Autodesk Fusion 360 part; units mm, degrees
(part 5 of 6)
  spline S16 degree 5 poles (-30.3241, -15.2327) (-30.3143, -15.242) (-30.2946, -15.2602) (-30.2642, -15.2865) (-30.2223, -15.3199) (-30.1678, -15.3592) (-30.1119, -15.3967) (-30.0551, -15.4332) (-29.9978, -15.4692) (-29.9401, -15.5048) (-29.8821, -15.5399) (-29.8236, -15.5744) (-29.7646, -15.6082) (-29.7048, -15.6412) (-29.6444, -15.6732) (-29.5834, -15.7045) (-29.5218, -15.735) (-29.4598, -15.765) (-29.3974, -15.7944) (-29.3347, -15.8233) (-29.2716, -15.8518) (-29.2081, -15.8797) (-29.1443, -15.907) (-29.08, -15.9338) (-29.0153, -15.96) (-28.9503, -15.9856) (-28.8849, -16.0108) (-28.8192, -16.0354) (-28.7532, -16.0595) (-28.6869, -16.0832) (-28.6202, -16.1064) (-28.5533, -16.1291) (-28.4861, -16.1513) (-28.4185, -16.1731) (-28.3507, -16.1943) (-28.2826, -16.2151) (-28.2142, -16.2355) (-28.1455, -16.2554) (-28.0766, -16.2748) (-28.0074, -16.2938) (-27.938, -16.3123) (-27.8683, -16.3304) (-27.7984, -16.3481) (-27.7282, -16.3653) (-27.6578, -16.3821) (-27.5872, -16.3984) (-27.5163, -16.4143) (-27.4452, -16.4298) (-27.3739, -16.4449) (-27.3024, -16.4595) (-27.2307, -16.4737) (-27.1587, -16.4875) (-27.0865, -16.5009) (-27.0142, -16.5139) (-26.9416, -16.5264) (-26.8689, -16.5386) (-26.7959, -16.5503) (-26.7228, -16.5616) (-26.6494, -16.5725) (-26.5759, -16.583) (-26.5022, -16.5931) (-26.4283, -16.6028) (-26.3543, -16.6121) (-26.2801, -16.621) (-26.2057, -16.6295) (-26.1311, -16.6376) (-26.0564, -16.6453) (-25.9815, -16.6526) (-25.9065, -16.6595) (-25.8313, -16.666) (-25.7559, -16.6721) (-25.6955, -16.6767) (-25.6501, -16.68) (-25.6199, -16.6821) (-25.6047, -16.6831) knots 0 0 0 0 0 0 0.01428571 0.02857143 0.04285714 0.05714286 0.07142857 0.08571429 0.1 0.11428571 0.12857143 0.14285714 0.15714286 0.17142857 0.18571429 0.2 0.21428571 0.22857143 0.24285714 0.25714286 0.27142857 0.28571429 0.3 0.31428571 0.32857143 0.34285714 0.35714286 0.37142857 0.38571429 0.4 0.41428571 0.42857143 0.44285714 0.45714286 0.47142857 0.48571429 0.5 0.51428571 0.52857143 0.54285714 0.55714286 0.57142857 0.58571429 0.6 0.61428571 0.62857143 0.64285714 0.65714286 0.67142857 0.68571429 0.7 0.71428571 0.72857143 0.74285714 0.75714286 0.77142857 0.78571429 0.8 0.81428571 0.82857143 0.84285714 0.85714286 0.87142857 0.88571429 0.9 0.91428571 0.92857143 0.94285714 0.95714286 0.97142857 0.98571429 1 1 1 1 1 1
  arc A32 (-25.6047, -16.6831) -> (-24.4732, -15.15) centre (-45.4614, -0.8441) ccw
  spline S17 degree 5 poles (-24.4732, -15.15) (-24.4787, -15.1359) (-24.4896, -15.1075) (-24.5061, -15.0651) (-24.5283, -15.0088) (-24.5564, -14.9386) (-24.5847, -14.8686) (-24.6135, -14.799) (-24.6425, -14.7296) (-24.6719, -14.6604) (-24.7016, -14.5916) (-24.7317, -14.523) (-24.762, -14.4547) (-24.7927, -14.3866) (-24.8238, -14.3189) (-24.8552, -14.2515) (-24.8869, -14.1843) (-24.9189, -14.1175) (-24.9513, -14.0509) (-24.984, -13.9846) (-25.017, -13.9187) (-25.0504, -13.8531) (-25.0841, -13.7877) (-25.1182, -13.7227) (-25.1526, -13.658) (-25.1873, -13.5937) (-25.2224, -13.5296) (-25.2578, -13.4659) (-25.2935, -13.4025) (-25.3296, -13.3395) (-25.3661, -13.2768) (-25.4029, -13.2145) (-25.44, -13.1525) (-25.4775, -13.0909) (-25.5153, -13.0297) (-25.5535, -12.9688) (-25.592, -12.9083) (-25.6309, -12.8481) (-25.6701, -12.7884) (-25.7097, -12.729) (-25.7497, -12.6701) (-25.79, -12.6115) (-25.8307, -12.5534) (-25.8718, -12.4957) (-25.9132, -12.4385) (-25.955, -12.3816) (-25.9971, -12.3252) (-26.0397, -12.2692) (-26.0826, -12.2137) (-26.1259, -12.1586) (-26.1695, -12.1041) (-26.2136, -12.05) (-26.2582, -11.9965) (-26.3031, -11.9435) (-26.3485, -11.8911) (-26.3942, -11.8392) (-26.4404, -11.7878) (-26.4869, -11.7368) (-26.5338, -11.6864) (-26.5811, -11.6366) (-26.629, -11.5875) (-26.6774, -11.5392) (-26.7265, -11.4918) (-26.7762, -11.4453) (-26.8265, -11.3996) (-26.8771, -11.3546) (-26.9281, -11.3099) (-26.9793, -11.2658) (-27.031, -11.2222) (-27.0834, -11.1799) (-27.137, -11.1394) (-27.1812, -11.1092) (-27.2153, -11.0879) (-27.2385, -11.0744) (-27.2502, -11.0678) knots -1 -1 -1 -1 -1 -1 -0.98571429 -0.97142857 -0.95714286 -0.94285714 -0.92857143 -0.91428571 -0.9 -0.88571429 -0.87142857 -0.85714286 -0.84285714 -0.82857143 -0.81428571 -0.8 -0.78571429 -0.77142857 -0.75714286 -0.74285714 -0.72857143 -0.71428571 -0.7 -0.68571429 -0.67142857 -0.65714286 -0.64285714 -0.62857143 -0.61428571 -0.6 -0.58571429 -0.57142857 -0.55714286 -0.54285714 -0.52857143 -0.51428571 -0.5 -0.48571429 -0.47142857 -0.45714286 -0.44285714 -0.42857143 -0.41428571 -0.4 -0.38571429 -0.37142857 -0.35714286 -0.34285714 -0.32857143 -0.31428571 -0.3 -0.28571429 -0.27142857 -0.25714286 -0.24285714 -0.22857143 -0.21428571 -0.2 -0.18571429 -0.17142857 -0.15714286 -0.14285714 -0.12857143 -0.11428571 -0.1 -0.08571429 -0.07142857 -0.05714286 -0.04285714 -0.02857143 -0.01428571 0 0 0 0 0 0
  line L19 (-27.2502, -11.0678) -> (-28.1194, -10.5793)
  arc A33 (-28.7833, -8.5309) -> (-28.1194, -10.5793) centre (-27.3416, -9.1954) ccw
  arc A34 (-28.7833, -8.5309) -> (-28.4826, -7.8417) centre (-45.4614, -0.8441) ccw
  arc A35 (-26.5294, -6.9351) -> (-28.4826, -7.8417) centre (-27.0149, -8.4466) ccw
  line L20 (-26.5294, -6.9351) -> (-25.5802, -7.24)
  spline S18 degree 5 poles (-25.5802, -7.24) (-25.5674, -7.2441) (-25.5417, -7.2519) (-25.5029, -7.2625) (-25.4506, -7.2743) (-25.3845, -7.2861) (-25.3178, -7.2957) (-25.2508, -7.3039) (-25.1836, -7.3115) (-25.1162, -7.3185) (-25.0487, -7.325) (-24.981, -7.3307) (-24.9131, -7.3356) (-24.845, -7.3393) (-24.7767, -7.342) (-24.7081, -7.3436) (-24.6394, -7.3444) (-24.5705, -7.3445) (-24.5016, -7.344) (-24.4325, -7.3428) (-24.3633, -7.3411) (-24.294, -7.3387) (-24.2246, -7.3356) (-24.1551, -7.3318) (-24.0855, -7.3274) (-24.0158, -7.3223) (-23.946, -7.3165) (-23.8761, -7.3102) (-23.8061, -7.3033) (-23.7361, -7.2959) (-23.666, -7.2878) (-23.5958, -7.2793) (-23.5256, -7.2701) (-23.4553, -7.2604) (-23.385, -7.2501) (-23.3146, -7.2393) (-23.2442, -7.228) (-23.1737, -7.2161) (-23.1031, -7.2037) (-23.0326, -7.1908) (-22.962, -7.1774) (-22.8914, -7.1635) (-22.8207, -7.149) (-22.75, -7.1341) (-22.6793, -7.1187) (-22.6086, -7.1027) (-22.5378, -7.0863) (-22.467, -7.0694) (-22.3962, -7.0521) (-22.3254, -7.0342) (-22.2546, -7.0159) (-22.1838, -6.9971) (-22.113, -6.9779) (-22.0422, -6.9581) (-21.9714, -6.938) (-21.9005, -6.9173) (-21.8297, -6.8962) (-21.7589, -6.8747) (-21.6881, -6.8527) (-21.6173, -6.8303) (-21.5465, -6.8074) (-21.4758, -6.7841) (-21.405, -6.7603) (-21.3343, -6.7361) (-21.2636, -6.7115) (-21.1929, -6.6865) (-21.1222, -6.661) (-21.0516, -6.6351) (-20.981, -6.6087) (-20.9104, -6.582) (-20.8399, -6.5548) (-20.7834, -6.5327) (-20.7412, -6.516) (-20.713, -6.5047) (-20.6989, -6.4991) knots 0 0 0 0 0 0 0.01428571 0.02857143 0.04285714 0.05714286 0.07142857 0.08571429 0.1 0.11428571 0.12857143 0.14285714 0.15714286 0.17142857 0.18571429 0.2 0.21428571 0.22857143 0.24285714 0.25714286 0.27142857 0.28571429 0.3 0.31428571 0.32857143 0.34285714 0.35714286 0.37142857 0.38571429 0.4 0.41428571 0.42857143 0.44285714 0.45714286 0.47142857 0.48571429 0.5 0.51428571 0.52857143 0.54285714 0.55714286 0.57142857 0.58571429 0.6 0.61428571 0.62857143 0.64285714 0.65714286 0.67142857 0.68571429 0.7 0.71428571 0.72857143 0.74285714 0.75714286 0.77142857 0.78571429 0.8 0.81428571 0.82857143 0.84285714 0.85714286 0.87142857 0.88571429 0.9 0.91428571 0.92857143 0.94285714 0.95714286 0.97142857 0.98571429 1 1 1 1 1 1
  arc A36 (-20.6989, -6.4991) -> (-20.3446, -4.6269) centre (-45.4614, -0.8441) ccw
  spline S19 degree 5 poles (-20.3446, -4.6269) (-20.3557, -4.6165) (-20.3778, -4.5957) (-20.4111, -4.5647) (-20.4555, -4.5235) (-20.5113, -4.4724) (-20.5672, -4.4217) (-20.6233, -4.3714) (-20.6796, -4.3215) (-20.736, -4.272) (-20.7927, -4.2228) (-20.8495, -4.1741) (-20.9065, -4.1257) (-20.9637, -4.0777) (-21.0211, -4.0302) (-21.0786, -3.983) (-21.1363, -3.9363) (-21.1942, -3.8899) (-21.2522, -3.844) (-21.3104, -3.7985) (-21.3688, -3.7534) (-21.4274, -3.7088) (-21.4861, -3.6645) (-21.545, -3.6208) (-21.604, -3.5774) (-21.6633, -3.5345) (-21.7226, -3.492) (-21.7822, -3.45) (-21.8419, -3.4084) (-21.9018, -3.3673) (-21.9618, -3.3266) (-22.022, -3.2864) (-22.0823, -3.2467) (-22.1428, -3.2074) (-22.2035, -3.1686) (-22.2643, -3.1304) (-22.3253, -3.0926) (-22.3864, -3.0553) (-22.4477, -3.0185) (-22.5091, -2.9822) (-22.5707, -2.9464) (-22.6324, -2.9111) (-22.6943, -2.8764) (-22.7563, -2.8422) (-22.8185, -2.8086) (-22.8808, -2.7755) (-22.9433, -2.743) (-23.0059, -2.711) (-23.0686, -2.6796) (-23.1315, -2.6488) (-23.1945, -2.6186) (-23.2577, -2.589) (-23.3211, -2.5601) (-23.3845, -2.5319) (-23.4482, -2.5043) (-23.5119, -2.4774) (-23.5758, -2.4511) (-23.6398, -2.4254) (-23.7039, -2.4003) (-23.7682, -2.376) (-23.8326, -2.3525) (-23.8972, -2.33) (-23.962, -2.3086) (-24.0269, -2.2883) (-24.092, -2.2689) (-24.1572, -2.2503) (-24.2225, -2.2322) (-24.2879, -2.2147) (-24.3533, -2.1978) (-24.4189, -2.1824) (-24.4847, -2.1692) (-24.5377, -2.1611) (-24.5777, -2.1568) (-24.6044, -2.1547) (-24.6178, -2.1539) knots -1 -1 -1 -1 -1 -1 -0.98571429 -0.97142857 -0.95714286 -0.94285714 -0.92857143 -0.91428571 -0.9 -0.88571429 -0.87142857 -0.85714286 -0.84285714 -0.82857143 -0.81428571 -0.8 -0.78571429 -0.77142857 -0.75714286 -0.74285714 -0.72857143 -0.71428571 -0.7 -0.68571429 -0.67142857 -0.65714286 -0.64285714 -0.62857143 -0.61428571 -0.6 -0.58571429 -0.57142857 -0.55714286 -0.54285714 -0.52857143 -0.51428571 -0.5 -0.48571429 -0.47142857 -0.45714286 -0.44285714 -0.42857143 -0.41428571 -0.4 -0.38571429 -0.37142857 -0.35714286 -0.34285714 -0.32857143 -0.31428571 -0.3 -0.28571429 -0.27142857 -0.25714286 -0.24285714 -0.22857143 -0.21428571 -0.2 -0.18571429 -0.17142857 -0.15714286 -0.14285714 -0.12857143 -0.11428571 -0.1 -0.08571429 -0.07142857 -0.05714286 -0.04285714 -0.02857143 -0.01428571 0 0 0 0 0 0
  line L21 (-24.6178, -2.1539) -> (-25.6129, -2.0908)
  arc A37 (-27.0998, -0.5334) -> (-25.6129, -2.0908) centre (-25.5125, -0.5065) ccw
  arc A38 (-27.0998, -0.5334) -> (-27.1279, 0.2181) centre (-45.4614, -0.8441) ccw
  arc A39 (-25.7615, 1.8823) -> (-27.1279, 0.2181) centre (-25.5431, 0.31) ccw
  line L22 (-25.7615, 1.8823) -> (-24.774, 2.0195)
  spline S20 degree 5 poles (-24.774, 2.0195) (-24.7607, 2.0214) (-24.7342, 2.0255) (-24.6946, 2.0328) (-24.6424, 2.0448) (-24.5777, 2.0629) (-24.5135, 2.0832) (-24.4495, 2.1048) (-24.3856, 2.1272) (-24.3219, 2.1501) (-24.2583, 2.1736) (-24.1948, 2.1977) (-24.1315, 2.2228) (-24.0685, 2.249) (-24.0058, 2.2763) (-23.9433, 2.3045) (-23.8811, 2.3336) (-23.819, 2.3634) (-23.7571, 2.3938) (-23.6953, 2.4248) (-23.6338, 2.4564) (-23.5724, 2.4887) (-23.5112, 2.5216) (-23.4502, 2.5551) (-23.3894, 2.5893) (-23.3288, 2.6242) (-23.2684, 2.6596) (-23.2082, 2.6956) (-23.1481, 2.7322) (-23.0883, 2.7693) (-23.0286, 2.8069) (-22.9691, 2.8451) (-22.9098, 2.8838) (-22.8507, 2.9231) (-22.7918, 2.9628) (-22.7331, 3.0031) (-22.6745, 3.0439) (-22.6162, 3.0852) (-22.558, 3.127) (-22.5, 3.1692) (-22.4422, 3.2119) (-22.3846, 3.2551) (-22.3272, 3.2988) (-22.27, 3.3429) (-22.213, 3.3875) (-22.1562, 3.4325) (-22.0996, 3.478) (-22.0431, 3.5239) (-21.9869, 3.5703) (-21.9309, 3.6171) (-21.875, 3.6643) (-21.8194, 3.712) (-21.7639, 3.76) (-21.7086, 3.8085) (-21.6536, 3.8574) (-21.5987, 3.9068) (-21.5441, 3.9565) (-21.4896, 4.0066) (-21.4354, 4.0572) (-21.3813, 4.1081) (-21.3275, 4.1594) (-21.2739, 4.2111) (-21.2204, 4.2632) (-21.1672, 4.3157) (-21.1142, 4.3686) (-21.0613, 4.4218) (-21.0087, 4.4754) (-20.9563, 4.5294) (-20.9041, 4.5838) (-20.8522, 4.6385) (-20.8004, 4.6936) (-20.7592, 4.738) (-20.7283, 4.7714) (-20.7078, 4.7938) (-20.6975, 4.805) knots 0 0 0 0 0 0 0.01428571 0.02857143 0.04285714 0.05714286 0.07142857 0.08571429 0.1 0.11428571 0.12857143 0.14285714 0.15714286 0.17142857 0.18571429 0.2 0.21428571 0.22857143 0.24285714 0.25714286 0.27142857 0.28571429 0.3 0.31428571 0.32857143 0.34285714 0.35714286 0.37142857 0.38571429 0.4 0.41428571 0.42857143 0.44285714 0.45714286 0.47142857 0.48571429 0.5 0.51428571 0.52857143 0.54285714 0.55714286 0.57142857 0.58571429 0.6 0.61428571 0.62857143 0.64285714 0.65714286 0.67142857 0.68571429 0.7 0.71428571 0.72857143 0.74285714 0.75714286 0.77142857 0.78571429 0.8 0.81428571 0.82857143 0.84285714 0.85714286 0.87142857 0.88571429 0.9 0.91428571 0.92857143 0.94285714 0.95714286 0.97142857 0.98571429 1 1 1 1 1 1
  arc A40 (-20.6975, 4.805) -> (-21.1907, 6.6455) centre (-45.4614, -0.8441) ccw
  spline S21 degree 5 poles (-21.1907, 6.6455) (-21.2052, 6.65) (-21.2341, 6.6592) (-21.2776, 6.6727) (-21.3355, 6.6905) (-21.4078, 6.7123) (-21.4802, 6.7337) (-21.5526, 6.7547) (-21.625, 6.7753) (-21.6974, 6.7954) (-21.7697, 6.8151) (-21.8421, 6.8344) (-21.9144, 6.8532) (-21.9867, 6.8716) (-22.059, 6.8896) (-22.1313, 6.9071) (-22.2036, 6.9242) (-22.2759, 6.9408) (-22.3481, 6.957) (-22.4203, 6.9728) (-22.4924, 6.988) (-22.5646, 7.0029) (-22.6367, 7.0172) (-22.7087, 7.0312) (-22.7807, 7.0446) (-22.8527, 7.0576) (-22.9247, 7.0701) (-22.9965, 7.0821) (-23.0684, 7.0937) (-23.1402, 7.1047) (-23.2119, 7.1153) (-23.2836, 7.1254) (-23.3552, 7.135) (-23.4267, 7.1442) (-23.4982, 7.1528) (-23.5696, 7.1609) (-23.6409, 7.1685) (-23.7122, 7.1756) (-23.7833, 7.1821) (-23.8544, 7.1882) (-23.9254, 7.1937) (-23.9964, 7.1987) (-24.0672, 7.2031) (-24.1379, 7.207) (-24.2085, 7.2103) (-24.279, 7.2131) (-24.3494, 7.2153) (-24.4197, 7.2169) (-24.4898, 7.218) (-24.5599, 7.2185) (-24.6298, 7.2184) (-24.6995, 7.2176) (-24.7691, 7.2162) (-24.8385, 7.214) (-24.9078, 7.2113) (-24.9769, 7.2078) (-25.0459, 7.2038) (-25.1147, 7.1992) (-25.1834, 7.194) (-25.2519, 7.1881) (-25.3201, 7.1813) (-25.3881, 7.1735) (-25.4557, 7.1647) (-25.523, 7.1548) (-25.5901, 7.144) (-25.6569, 7.1325) (-25.7236, 7.1204) (-25.7901, 7.1079) (-25.8563, 7.0947) (-25.9221, 7.0801) (-25.9871, 7.0634) (-26.0384, 7.0477) (-26.0763, 7.0343) (-26.1013, 7.0246) (-26.1137, 7.0195) knots -1 -1 -1 -1 -1 -1 -0.98571429 -0.97142857 -0.95714286 -0.94285714 -0.92857143 -0.91428571 -0.9 -0.88571429 -0.87142857 -0.85714286 -0.84285714 -0.82857143 -0.81428571 -0.8 -0.78571429 -0.77142857 -0.75714286 -0.74285714 -0.72857143 -0.71428571 -0.7 -0.68571429 -0.67142857 -0.65714286 -0.64285714 -0.62857143 -0.61428571 -0.6 -0.58571429 -0.57142857 -0.55714286 -0.54285714 -0.52857143 -0.51428571 -0.5 -0.48571429 -0.47142857 -0.45714286 -0.44285714 -0.42857143 -0.41428571 -0.4 -0.38571429 -0.37142857 -0.35714286 -0.34285714 -0.32857143 -0.31428571 -0.3 -0.28571429 -0.27142857 -0.25714286 -0.24285714 -0.22857143 -0.21428571 -0.2 -0.18571429 -0.17142857 -0.15714286 -0.14285714 -0.12857143 -0.11428571 -0.1 -0.08571429 -0.07142857 -0.05714286 -0.04285714 -0.02857143 -0.01428571 0 0 0 0 0 0
  line L23 (-26.1137, 7.0195) -> (-27.0376, 6.6446)
  arc A41 (-29.053, 7.4026) -> (-27.0376, 6.6446) centre (-27.6346, 8.1155) ccw
  arc A42 (-29.053, 7.4026) -> (-29.4044, 8.0675) centre (-45.4614, -0.8441) ccw
  arc A43 (-28.8954, 10.1598) -> (-29.4044, 8.0675) centre (-28.0164, 8.8379) ccw
  line L24 (-28.8954, 10.1598) -> (-28.0652, 10.7119)
  spline S22 degree 5 poles (-28.0652, 10.7119) (-28.054, 10.7193) (-28.0319, 10.7345) (-27.9994, 10.7582) (-27.9576, 10.7917) (-27.9071, 10.8361) (-27.8581, 10.8822) (-27.8098, 10.9295) (-27.762, 10.9774) (-27.7145, 11.0257) (-27.6674, 11.0744) (-27.6207, 11.1237) (-27.5746, 11.1738) (-27.5292, 11.2247) (-27.4845, 11.2765) (-27.4404, 11.329) (-27.397, 11.3823) (-27.354, 11.4361) (-27.3114, 11.4903) (-27.2692, 11.545) (-27.2275, 11.6002) (-27.1861, 11.6559) (-27.1453, 11.7121) (-27.1049, 11.7688) (-27.0649, 11.826) (-27.0255, 11.8837) (-26.9864, 11.9418) (-26.9478, 12.0004) (-26.9096, 12.0594) (-26.8717, 12.1188) (-26.8343, 12.1786) (-26.7973, 12.2388) (-26.7606, 12.2994) (-26.7244, 12.3604) (-26.6886, 12.4218) (-26.6531, 12.4836) (-26.6181, 12.5457) (-26.5834, 12.6082) (-26.5491, 12.6711) (-26.5152, 12.7343) (-26.4817, 12.7979) (-26.4486, 12.8618) (-26.4158, 12.926) (-26.3834, 12.9906) (-26.3514, 13.0555) (-26.3197, 13.1207) (-26.2884, 13.1863) (-26.2575, 13.2522) (-26.227, 13.3183) (-26.1968, 13.3848) (-26.1669, 13.4516) (-26.1375, 13.5187) (-26.1084, 13.586) (-26.0796, 13.6537) (-26.0513, 13.7217) (-26.0232, 13.7899) (-25.9956, 13.8584) (-25.9683, 13.9272) (-25.9413, 13.9963) (-25.9147, 14.0656) (-25.8885, 14.1352) (-25.8626, 14.2051) (-25.837, 14.2752) (-25.8118, 14.3456) (-25.787, 14.4162) (-25.7625, 14.4871) (-25.7384, 14.5582) (-25.7146, 14.6296) (-25.6912, 14.7012) (-25.6681, 14.7731) (-25.6454, 14.8452) (-25.6274, 14.9031) (-25.6142, 14.9466) (-25.6054, 14.9756) (-25.601, 14.9902) knots 0 0 0 0 0 0 0.01428571 0.02857143 0.04285714 0.05714286 0.07142857 0.08571429 0.1 0.11428571 0.12857143 0.14285714 0.15714286 0.17142857 0.18571429 0.2 0.21428571 0.22857143 0.24285714 0.25714286 0.27142857 0.28571429 0.3 0.31428571 0.32857143 0.34285714 0.35714286 0.37142857 0.38571429 0.4 0.41428571 0.42857143 0.44285714 0.45714286 0.47142857 0.48571429 0.5 0.51428571 0.52857143 0.54285714 0.55714286 0.57142857 0.58571429 0.6 0.61428571 0.62857143 0.64285714 0.65714286 0.67142857 0.68571429 0.7 0.71428571 0.72857143 0.74285714 0.75714286 0.77142857 0.78571429 0.8 0.81428571 0.82857143 0.84285714 0.85714286 0.87142857 0.88571429 0.9 0.91428571 0.92857143 0.94285714 0.95714286 0.97142857 0.98571429 1 1 1 1 1 1
  arc A44 (-25.601, 14.9902) -> (-26.8439, 16.4344) centre (-45.4614, -0.8441) ccw
  spline S23 degree 5 poles (-26.8439, 16.4344) (-26.8589, 16.4323) (-26.8889, 16.4279) (-26.9339, 16.4213) (-26.9938, 16.4122) (-27.0685, 16.4004) (-27.143, 16.3883) (-27.2173, 16.3758) (-27.2915, 16.3629) (-27.3654, 16.3497) (-27.4392, 16.336) (-27.5127, 16.322) (-27.5861, 16.3076) (-27.6592, 16.2928) (-27.7322, 16.2776) (-27.8049, 16.262) (-27.8774, 16.2461) (-27.9497, 16.2297) (-28.0218, 16.213) (-28.0937, 16.1958) (-28.1653, 16.1783) (-28.2368, 16.1603) (-28.308, 16.142) (-28.3789, 16.1233) (-28.4496, 16.1041) (-28.5201, 16.0846) (-28.5903, 16.0646) (-28.6603, 16.0443) (-28.7301, 16.0235) (-28.7996, 16.0024) (-28.8688, 15.9808) (-28.9377, 15.9588) (-29.0064, 15.9364) (-29.0748, 15.9135) (-29.143, 15.8903) (-29.2108, 15.8666) (-29.2784, 15.8425) (-29.3456, 15.818) (-29.4126, 15.793) (-29.4793, 15.7676) (-29.5457, 15.7418) (-29.6117, 15.7155) (-29.6774, 15.6888) (-29.7428, 15.6616) (-29.8079, 15.634) (-29.8726, 15.6059) (-29.937, 15.5773) (-30.001, 15.5483) (-30.0647, 15.5188) (-30.128, 15.4889) (-30.1909, 15.4584) (-30.2535, 15.4275) (-30.3155, 15.396) (-30.3772, 15.3639) (-30.4384, 15.3314) (-30.4992, 15.2983) (-30.5596, 15.2648) (-30.6196, 15.2307) (-30.6792, 15.1962) (-30.7383, 15.1612) (-30.7968, 15.1255) (-30.8547, 15.089) (-30.9118, 15.0517) (-30.9682, 15.0136) (-31.0239, 14.9747) (-31.0791, 14.9354) (-31.1339, 14.8956) (-31.1884, 14.8555) (-31.2423, 14.8148) (-31.2953, 14.7732) (-31.3467, 14.7299) (-31.386, 14.6935) (-31.4143, 14.665) (-31.4326, 14.6454) (-31.4417, 14.6354) knots -1 -1 -1 -1 -1 -1 -0.98571429 -0.97142857 -0.95714286 -0.94285714 -0.92857143 -0.91428571 -0.9 -0.88571429 -0.87142857 -0.85714286 -0.84285714 -0.82857143 -0.81428571 -0.8 -0.78571429 -0.77142857 -0.75714286 -0.74285714 -0.72857143 -0.71428571 -0.7 -0.68571429 -0.67142857 -0.65714286 -0.64285714 -0.62857143 -0.61428571 -0.6 -0.58571429 -0.57142857 -0.55714286 -0.54285714 -0.52857143 -0.51428571 -0.5 -0.48571429 -0.47142857 -0.45714286 -0.44285714 -0.42857143 -0.41428571 -0.4 -0.38571429 -0.37142857 -0.35714286 -0.34285714 -0.32857143 -0.31428571 -0.3 -0.28571429 -0.27142857 -0.25714286 -0.24285714 -0.22857143 -0.21428571 -0.2 -0.18571429 -0.17142857 -0.15714286 -0.14285714 -0.12857143 -0.11428571 -0.1 -0.08571429 -0.07142857 -0.05714286 -0.04285714 -0.02857143 -0.01428571 0 0 0 0 0 0
  line L25 (-31.4417, 14.6354) -> (-32.1113, 13.8967)
  arc A45 (-34.2561, 13.7053) -> (-32.1113, 13.8967) centre (-33.2874, 14.963) ccw
  arc A46 (-34.2561, 13.7053) -> (-34.8612, 14.1518) centre (-45.4614, -0.8441) ccw
  arc A47 (-35.3981, 14.8093) -> (-34.8612, 14.1518) centre (-33.9448, 15.4482) ccw
  line L26 (-35.3981, 14.8093) -> (-33.2667, 19.4605)
  line L27 (-33.2667, 19.4605) -> (-34.2844, 20.5142)
  spline S24 degree 5 poles (-34.2844, 20.5142) (-34.2847, 20.5222) (-34.2856, 20.5448) (-34.2873, 20.5821) (-34.2898, 20.6341) (-34.2933, 20.7009) (-34.2977, 20.7746) (-34.3025, 20.8483) (-34.3077, 20.9221) (-34.3134, 20.996) (-34.3195, 21.0701) (-34.3261, 21.1441) (-34.3331, 21.2183) (-34.3405, 21.2926) (-34.3483, 21.3669) (-34.3566, 21.4413) (-34.3653, 21.5158) (-34.3744, 21.5904) (-34.384, 21.665) (-34.3939, 21.7397) (-34.4043, 21.8145) (-34.4151, 21.8893) (-34.4241, 21.9492) (-34.431, 21.9942) (-34.4357, 22.0242) (-34.4381, 22.0392) knots 0.70654 0.70654 0.70654 0.70654 0.70654 0.70654 0.714286 0.728571 0.742857 0.757143 0.771429 0.785714 0.8 0.814286 0.828571 0.842857 0.857143 0.871429 0.885714 0.9 0.914286 0.928571 0.942857 0.957143 0.971429 0.985714 1 1 1 1 1 1
  arc A48 (-34.4381, 22.0392) -> (-36.1845, 22.8011) centre (-45.4614, -0.8441) ccw
  spline S25 degree 5 poles (-36.1845, 22.8011) (-36.1971, 22.7927) (-36.2223, 22.7757) (-36.2596, 22.7504) (-36.2968, 22.725) (-36.3338, 22.6995) (-36.3583, 22.6825) (-36.3704, 22.6741) knots -1 -1 -1 -1 -1 -1 -0.985714 -0.971429 -0.957523 -0.957523 -0.957523 -0.957523 -0.957523 -0.957523
  line L28 (-36.3704, 22.6741) -> (-49.1726, 35.9298)
  line L29 (-49.1726, 35.9298) -> (-55.9036, 35.9298)
  line L30 (-49.1726, 17.3449) -> (-49.1726, 18.5703)
  line L31 (-49.1726, 18.5703) -> (-48.6457, 18.4228)
  arc A49 (-49.1726, 17.3449) -> (-48.6457, 18.4228) centre (-50.2296, 18.5294) ccw
  circle A50 centre (-45.4614, -0.8441) radius 3.175
  dimension "d39" = 6.35
  constraint concentric A0 A50
  measures "d39" diameter of A50
extrude "Extrude6" cut sketch "Sketch15" against normal blind 15.24 contours A50 sketch seen with x (0.965926, -0.258819, 0) y (0.258819, 0.965926, 0) z (0, 0, 1) at (44.1308, -10.9509, 0) bodies 2 in component "Spur Gear (14 teeth) (1)"
sketch "Sketch16" plane through (0, 0, 12.7) normal (0, 0, 1) x (1, 0, 0)
  circle A0 centre (-45.4614, -0.8441) radius 3.175
  line L0 (-55.9036, 35.9298) -> (-55.9036, 101.81)
  line L1 (-55.9036, 101.81) -> (-55.9735, 101.81)
  line L2 (-55.9735, 101.81) -> (-55.9735, 21.7403)
  spline S0 degree 5 poles (-55.9735, 21.7403) (-55.9837, 21.7467) (-56.0067, 21.761) (-56.0426, 21.7832) (-56.0913, 21.8132) (-56.1531, 21.8508) (-56.2177, 21.8896) (-56.2826, 21.928) (-56.3479, 21.9663) (-56.4003, 21.9966) (-56.4398, 22.0192) (-56.4661, 22.0343) (-56.4794, 22.0418) knots 0.888467 0.888467 0.888467 0.888467 0.888467 0.888467 0.9 0.914286 0.928571 0.942857 0.957143 0.971429 0.985714 1 1 1 1 1 1
  arc A1 (-56.4794, 22.0418) -> (-58.1639, 21.1514) centre (-45.4614, -0.8441) ccw
  spline S1 degree 5 poles (-58.1639, 21.1514) (-58.1652, 21.1363) (-58.1676, 21.106) (-58.1712, 21.0607) (-58.1756, 21.0003) (-58.1808, 20.9248) (-58.1856, 20.8495) (-58.1899, 20.7743) (-58.1939, 20.6991) (-58.1974, 20.6241) (-58.2005, 20.5492) (-58.2032, 20.4743) (-58.2055, 20.3996) (-58.2073, 20.325) (-58.2087, 20.2505) (-58.2097, 20.1761) (-58.2103, 20.1019) (-58.2104, 20.0277) (-58.2101, 19.9537) (-58.2094, 19.8798) (-58.2083, 19.8061) (-58.2067, 19.7325) (-58.2046, 19.659) (-58.2022, 19.5856) (-58.1992, 19.5124) (-58.1959, 19.4394) (-58.1921, 19.3665) (-58.1878, 19.2937) (-58.1831, 19.2211) (-58.1779, 19.1486) (-58.1723, 19.0763) (-58.1662, 19.0042) (-58.1596, 18.9323) (-58.1526, 18.8605) (-58.1451, 18.7889) (-58.1371, 18.7175) (-58.1286, 18.6463) (-58.1197, 18.5752) (-58.1102, 18.5044) (-58.1003, 18.4337) (-58.0899, 18.3632) (-58.079, 18.293) (-58.0675, 18.223) (-58.0556, 18.1532) (-58.0431, 18.0836) (-58.0301, 18.0143) (-58.0166, 17.9451) (-58.0026, 17.8763) (-57.988, 17.8076) (-57.9729, 17.7392) (-57.9572, 17.6711) (-57.941, 17.6033) (-57.9241, 17.5357) (-57.9065, 17.4685) (-57.8884, 17.4016) (-57.8697, 17.335) (-57.8504, 17.2686) (-57.8306, 17.2025) (-57.8103, 17.1368) (-57.7892, 17.0713) (-57.7674, 17.0063) (-57.7447, 16.9418) (-57.7211, 16.8778) (-57.6965, 16.8144) (-57.671, 16.7514) (-57.6449, 16.6888) (-57.6183, 16.6265) (-57.5913, 16.5645) (-57.5637, 16.5029) (-57.5349, 16.442) (-57.5041, 16.3822) (-57.4774, 16.3358) (-57.4559, 16.3018) (-57.4408, 16.2796) (-57.4332, 16.2686) knots -1 -1 -1 -1 -1 -1 -0.98571429 -0.97142857 -0.95714286 -0.94285714 -0.92857143 -0.91428571 -0.9 -0.88571429 -0.87142857 -0.85714286 -0.84285714 -0.82857143 -0.81428571 -0.8 -0.78571429 -0.77142857 -0.75714286 -0.74285714 -0.72857143 -0.71428571 -0.7 -0.68571429 -0.67142857 -0.65714286 -0.64285714 -0.62857143 -0.61428571 -0.6 -0.58571429 -0.57142857 -0.55714286 -0.54285714 -0.52857143 -0.51428571 -0.5 -0.48571429 -0.47142857 -0.45714286 -0.44285714 -0.42857143 -0.41428571 -0.4 -0.38571429 -0.37142857 -0.35714286 -0.34285714 -0.32857143 -0.31428571 -0.3 -0.28571429 -0.27142857 -0.25714286 -0.24285714 -0.22857143 -0.21428571 -0.2 -0.18571429 -0.17142857 -0.15714286 -0.14285714 -0.12857143 -0.11428571 -0.1 -0.08571429 -0.07142857 -0.05714286 -0.04285714 -0.02857143 -0.01428571 0 0 0 0 0 0
  line L3 (-57.4332, 16.2686) -> (-56.862, 15.4514)
  arc A2 (-57.1526, 13.3178) -> (-56.862, 15.4514) centre (-58.1632, 14.542) ccw
  arc A3 (-57.1526, 13.3178) -> (-57.7226, 12.8272) centre (-45.4614, -0.8441) ccw
  arc A4 (-59.8757, 12.8579) -> (-57.7226, 12.8272) centre (-58.7825, 14.009) ccw
  line L4 (-59.8757, 12.8579) -> (-60.5987, 13.5444)
  spline S2 degree 5 poles (-60.5987, 13.5444) (-60.6084, 13.5537) (-60.6281, 13.5719) (-60.6585, 13.5982) (-60.7005, 13.6316) (-60.7549, 13.6709) (-60.8109, 13.7084) (-60.8677, 13.745) (-60.925, 13.7809) (-60.9826, 13.8165) (-61.0407, 13.8516) (-61.0991, 13.8862) (-61.1582, 13.92) (-61.2179, 13.9529) (-61.2783, 13.9849) (-61.3394, 14.0162) (-61.401, 14.0467) (-61.463, 14.0767) (-61.5253, 14.1061) (-61.5881, 14.135) (-61.6512, 14.1635) (-61.7146, 14.1914) (-61.7785, 14.2187) (-61.8428, 14.2455) (-61.9074, 14.2717) (-61.9724, 14.2973) (-62.0378, 14.3225) (-62.1035, 14.3471) (-62.1695, 14.3712) (-62.2359, 14.3949) (-62.3025, 14.4181) (-62.3695, 14.4408) (-62.4367, 14.463) (-62.5042, 14.4848) (-62.5721, 14.506) (-62.6402, 14.5268) (-62.7086, 14.5472) (-62.7772, 14.5671) (-62.8461, 14.5865) (-62.9153, 14.6055) (-62.9847, 14.624) (-63.0544, 14.6421) (-63.1243, 14.6598) (-63.1945, 14.677) (-63.2649, 14.6938) (-63.3356, 14.7101) (-63.4064, 14.726) (-63.4775, 14.7415) (-63.5488, 14.7566) (-63.6204, 14.7712) (-63.6921, 14.7854) (-63.7641, 14.7992) (-63.8362, 14.8126) (-63.9086, 14.8256) (-63.9811, 14.8381) (-64.0539, 14.8503) (-64.1269, 14.862) (-64.2, 14.8733) (-64.2733, 14.8842) (-64.3468, 14.8947) (-64.4205, 14.9048) (-64.4944, 14.9145) (-64.5685, 14.9238) (-64.6427, 14.9327) (-64.7171, 14.9412) (-64.7916, 14.9493) (-64.8664, 14.957) (-64.9412, 14.9643) (-65.0163, 14.9712) (-65.0915, 14.9777) (-65.1668, 14.9838) (-65.2272, 14.9884) (-65.2726, 14.9917) (-65.3029, 14.9938) (-65.318, 14.9948) knots 0 0 0 0 0 0 0.01428571 0.02857143 0.04285714 0.05714286 0.07142857 0.08571429 0.1 0.11428571 0.12857143 0.14285714 0.15714286 0.17142857 0.18571429 0.2 0.21428571 0.22857143 0.24285714 0.25714286 0.27142857 0.28571429 0.3 0.31428571 0.32857143 0.34285714 0.35714286 0.37142857 0.38571429 0.4 0.41428571 0.42857143 0.44285714 0.45714286 0.47142857 0.48571429 0.5 0.51428571 0.52857143 0.54285714 0.55714286 0.57142857 0.58571429 0.6 0.61428571 0.62857143 0.64285714 0.65714286 0.67142857 0.68571429 0.7 0.71428571 0.72857143 0.74285714 0.75714286 0.77142857 0.78571429 0.8 0.81428571 0.82857143 0.84285714 0.85714286 0.87142857 0.88571429 0.9 0.91428571 0.92857143 0.94285714 0.95714286 0.97142857 0.98571429 1 1 1 1 1 1
  arc A5 (-65.318, 14.9948) -> (-66.4495, 13.4617) centre (-45.4614, -0.8441) ccw
  spline S3 degree 5 poles (-66.4495, 13.4617) (-66.4441, 13.4476) (-66.4331, 13.4192) (-66.4166, 13.3768) (-66.3945, 13.3205) (-66.3664, 13.2503) (-66.338, 13.1803) (-66.3093, 13.1107) (-66.2802, 13.0413) (-66.2509, 12.9721) (-66.2211, 12.9033) (-66.1911, 12.8347) (-66.1607, 12.7664) (-66.13, 12.6984) (-66.099, 12.6306) (-66.0676, 12.5632) (-66.0359, 12.496) (-66.0039, 12.4292) (-65.9715, 12.3626) (-65.9388, 12.2964) (-65.9057, 12.2304) (-65.8723, 12.1648) (-65.8386, 12.0994) (-65.8046, 12.0344) (-65.7702, 11.9697) (-65.7354, 11.9054) (-65.7004, 11.8413) (-65.665, 11.7776) (-65.6292, 11.7143) (-65.5931, 11.6512) (-65.5567, 11.5885) (-65.5199, 11.5262) (-65.4828, 11.4642) (-65.4453, 11.4026) (-65.4074, 11.3414) (-65.3693, 11.2805) (-65.3307, 11.22) (-65.2918, 11.1599) (-65.2526, 11.1001) (-65.213, 11.0408) (-65.1731, 10.9818) (-65.1327, 10.9233) (-65.0921, 10.8651) (-65.051, 10.8074) (-65.0096, 10.7502) (-64.9678, 10.6933) (-64.9256, 10.6369) (-64.8831, 10.5809) (-64.8402, 10.5254) (-64.7969, 10.4703) (-64.7532, 10.4158) (-64.7091, 10.3617) (-64.6646, 10.3082) (-64.6196, 10.2552) (-64.5743, 10.2028) (-64.5285, 10.1509) (-64.4824, 10.0995) (-64.4359, 10.0485) (-64.389, 9.9981) (-64.3416, 9.9483) (-64.2938, 9.8992) (-64.2453, 9.8509) (-64.1963, 9.8035) (-64.1466, 9.757) (-64.0963, 9.7113) (-64.0456, 9.6663) (-63.9947, 9.6217) (-63.9434, 9.5775) (-63.8918, 9.534) (-63.8394, 9.4916) (-63.7858, 9.4511) (-63.7415, 9.4209) (-63.7074, 9.3996) (-63.6842, 9.3861) (-63.6725, 9.3795) knots -1 -1 -1 -1 -1 -1 -0.98571429 -0.97142857 -0.95714286 -0.94285714 -0.92857143 -0.91428571 -0.9 -0.88571429 -0.87142857 -0.85714286 -0.84285714 -0.82857143 -0.81428571 -0.8 -0.78571429 -0.77142857 -0.75714286 -0.74285714 -0.72857143 -0.71428571 -0.7 -0.68571429 -0.67142857 -0.65714286 -0.64285714 -0.62857143 -0.61428571 -0.6 -0.58571429 -0.57142857 -0.55714286 -0.54285714 -0.52857143 -0.51428571 -0.5 -0.48571429 -0.47142857 -0.45714286 -0.44285714 -0.42857143 -0.41428571 -0.4 -0.38571429 -0.37142857 -0.35714286 -0.34285714 -0.32857143 -0.31428571 -0.3 -0.28571429 -0.27142857 -0.25714286 -0.24285714 -0.22857143 -0.21428571 -0.2 -0.18571429 -0.17142857 -0.15714286 -0.14285714 -0.12857143 -0.11428571 -0.1 -0.08571429 -0.07142857 -0.05714286 -0.04285714 -0.02857143 -0.01428571 0 0 0 0 0 0
  line L5 (-63.6725, 9.3795) -> (-62.8034, 8.891)
  arc A6 (-62.1394, 6.8427) -> (-62.8034, 8.891) centre (-63.5812, 7.5071) ccw
  arc A7 (-62.1394, 6.8427) -> (-62.4401, 6.1534) centre (-45.4614, -0.8441) ccw
  arc A8 (-64.3933, 5.2468) -> (-62.4401, 6.1534) centre (-63.9079, 6.7583) ccw
  line L6 (-64.3933, 5.2468) -> (-65.3426, 5.5517)
  spline S4 degree 5 poles (-65.3426, 5.5517) (-65.3554, 5.5558) (-65.381, 5.5636) (-65.4198, 5.5742) (-65.4721, 5.586) (-65.5382, 5.5978) (-65.6049, 5.6074) (-65.672, 5.6156) (-65.7392, 5.6232) (-65.8066, 5.6302) (-65.8741, 5.6367) (-65.9417, 5.6424) (-66.0096, 5.6473) (-66.0777, 5.651) (-66.1461, 5.6537) (-66.2146, 5.6553) (-66.2833, 5.6561) (-66.3522, 5.6562) (-66.4212, 5.6557) (-66.4903, 5.6545) (-66.5594, 5.6528) (-66.6287, 5.6504) (-66.6981, 5.6473) (-66.7676, 5.6435) (-66.8373, 5.6391) (-66.907, 5.634) (-66.9768, 5.6283) (-67.0467, 5.6219) (-67.1166, 5.615) (-67.1867, 5.6076) (-67.2568, 5.5996) (-67.3269, 5.591) (-67.3971, 5.5818) (-67.4674, 5.5721) (-67.5378, 5.5619) (-67.6082, 5.551) (-67.6786, 5.5397) (-67.7491, 5.5278) (-67.8196, 5.5154) (-67.8902, 5.5025) (-67.9608, 5.4891) (-68.0314, 5.4752) (-68.1021, 5.4607) (-68.1727, 5.4458) (-68.2435, 5.4304) (-68.3142, 5.4145) (-68.3849, 5.398) (-68.4557, 5.3811) (-68.5265, 5.3638) (-68.5973, 5.3459) (-68.6681, 5.3276) (-68.7389, 5.3088) (-68.8097, 5.2896) (-68.8806, 5.2699) (-68.9514, 5.2497) (-69.0222, 5.229) (-69.093, 5.208) (-69.1638, 5.1864) (-69.2346, 5.1644) (-69.3054, 5.142) (-69.3762, 5.1191) (-69.447, 5.0958) (-69.5177, 5.072) (-69.5885, 5.0479) (-69.6592, 5.0232) (-69.7299, 4.9982) (-69.8005, 4.9727) (-69.8712, 4.9468) (-69.9418, 4.9204) (-70.0123, 4.8937) (-70.0829, 4.8665) (-70.1393, 4.8444) (-70.1816, 4.8277) (-70.2098, 4.8164) (-70.2239, 4.8108) knots 0 0 0 0 0 0 0.01428571 0.02857143 0.04285714 0.05714286 0.07142857 0.08571429 0.1 0.11428571 0.12857143 0.14285714 0.15714286 0.17142857 0.18571429 0.2 0.21428571 0.22857143 0.24285714 0.25714286 0.27142857 0.28571429 0.3 0.31428571 0.32857143 0.34285714 0.35714286 0.37142857 0.38571429 0.4 0.41428571 0.42857143 0.44285714 0.45714286 0.47142857 0.48571429 0.5 0.51428571 0.52857143 0.54285714 0.55714286 0.57142857 0.58571429 0.6 0.61428571 0.62857143 0.64285714 0.65714286 0.67142857 0.68571429 0.7 0.71428571 0.72857143 0.74285714 0.75714286 0.77142857 0.78571429 0.8 0.81428571 0.82857143 0.84285714 0.85714286 0.87142857 0.88571429 0.9 0.91428571 0.92857143 0.94285714 0.95714286 0.97142857 0.98571429 1 1 1 1 1 1
  arc A9 (-70.2239, 4.8108) -> (-70.5781, 2.9386) centre (-45.4614, -0.8441) ccw
  spline S5 degree 5 poles (-70.5781, 2.9386) (-70.5671, 2.9282) (-70.5449, 2.9074) (-70.5117, 2.8764) (-70.4672, 2.8352) (-70.4115, 2.7841) (-70.3556, 2.7334) (-70.2995, 2.6831) (-70.2432, 2.6332) (-70.1867, 2.5837) (-70.1301, 2.5345) (-70.0732, 2.4858) (-70.0162, 2.4374) (-69.959, 2.3894) (-69.9017, 2.3419) (-69.8442, 2.2947) (-69.7865, 2.248) (-69.7286, 2.2016) (-69.6705, 2.1557) (-69.6123, 2.1102) (-69.5539, 2.0651) (-69.4954, 2.0205) (-69.4367, 1.9763) (-69.3778, 1.9325) (-69.3187, 1.8891) (-69.2595, 1.8462) (-69.2001, 1.8037) (-69.1406, 1.7617) (-69.0809, 1.7201) (-69.021, 1.679) (-68.961, 1.6383) (-68.9008, 1.5981) (-68.8404, 1.5584) (-68.7799, 1.5191) (-68.7193, 1.4804) (-68.6584, 1.4421) (-68.5975, 1.4043) (-68.5364, 1.367) (-68.4751, 1.3302) (-68.4137, 1.2939) (-68.3521, 1.2581) (-68.2903, 1.2228) (-68.2285, 1.1881) (-68.1664, 1.1539) (-68.1043, 1.1203) (-68.0419, 1.0873) (-67.9795, 1.0547) (-67.9169, 1.0227) (-67.8541, 0.9913) (-67.7912, 0.9605) (-67.7282, 0.9303) (-67.665, 0.9007) (-67.6017, 0.8718) (-67.5382, 0.8436) (-67.4746, 0.816) (-67.4108, 0.7891) (-67.347, 0.7628) (-67.2829, 0.7371) (-67.2188, 0.712) (-67.1546, 0.6877) (-67.0901, 0.6642) (-67.0255, 0.6417) (-66.9608, 0.6203) (-66.8958, 0.6) (-66.8307, 0.5806) (-66.7655, 0.562) (-66.7002, 0.5439) (-66.6349, 0.5264) (-66.5695, 0.5096) (-66.5039, 0.4941) (-66.438, 0.4809) (-66.3851, 0.4729) (-66.3451, 0.4685) (-66.3183, 0.4664) (-66.3049, 0.4656) knots -1 -1 -1 -1 -1 -1 -0.98571429 -0.97142857 -0.95714286 -0.94285714 -0.92857143 -0.91428571 -0.9 -0.88571429 -0.87142857 -0.85714286 -0.84285714 -0.82857143 -0.81428571 -0.8 -0.78571429 -0.77142857 -0.75714286 -0.74285714 -0.72857143 -0.71428571 -0.7 -0.68571429 -0.67142857 -0.65714286 -0.64285714 -0.62857143 -0.61428571 -0.6 -0.58571429 -0.57142857 -0.55714286 -0.54285714 -0.52857143 -0.51428571 -0.5 -0.48571429 -0.47142857 -0.45714286 -0.44285714 -0.42857143 -0.41428571 -0.4 -0.38571429 -0.37142857 -0.35714286 -0.34285714 -0.32857143 -0.31428571 -0.3 -0.28571429 -0.27142857 -0.25714286 -0.24285714 -0.22857143 -0.21428571 -0.2 -0.18571429 -0.17142857 -0.15714286 -0.14285714 -0.12857143 -0.11428571 -0.1 -0.08571429 -0.07142857 -0.05714286 -0.04285714 -0.02857143 -0.01428571 0 0 0 0 0 0
  line L7 (-66.3049, 0.4656) -> (-65.3099, 0.4026)
  arc A10 (-63.8229, -1.1549) -> (-65.3099, 0.4026) centre (-65.4102, -1.1818) ccw
  arc A11 (-63.8229, -1.1549) -> (-63.7948, -1.9064) centre (-45.4614, -0.8441) ccw
  arc A12 (-65.1612, -3.5706) -> (-63.7948, -1.9064) centre (-65.3797, -1.9982) ccw
  line L8 (-65.1612, -3.5706) -> (-66.1488, -3.7078)
  spline S6 degree 5 poles (-66.1488, -3.7078) (-66.1621, -3.7097) (-66.1886, -3.7138) (-66.2281, -3.7211) (-66.2804, -3.7331) (-66.3451, -3.7512) (-66.4093, -3.7715) (-66.4733, -3.7931) (-66.5371, -3.8155) (-66.6009, -3.8384) (-66.6645, -3.8619) (-66.728, -3.886) (-66.7912, -3.9111) (-66.8542, -3.9373) (-66.9169, -3.9646) (-66.9794, -3.9928) (-67.0417, -4.0219) (-67.1038, -4.0517) (-67.1657, -4.0821) (-67.2274, -4.1131) (-67.289, -4.1447) (-67.3504, -4.177) (-67.4116, -4.2098) (-67.4725, -4.2434) (-67.5333, -4.2776) (-67.5939, -4.3124) (-67.6544, -4.3479) (-67.7146, -4.3839) (-67.7746, -4.4205) (-67.8345, -4.4576) (-67.8942, -4.4952) (-67.9536, -4.5334) (-68.0129, -4.5721) (-68.072, -4.6114) (-68.131, -4.6511) (-68.1897, -4.6914) (-68.2482, -4.7322) (-68.3066, -4.7735) (-68.3648, -4.8152) (-68.4227, -4.8575) (-68.4805, -4.9002) (-68.5381, -4.9434) (-68.5955, -4.9871) (-68.6527, -5.0312) (-68.7097, -5.0758) (-68.7666, -5.1208) (-68.8232, -5.1663) (-68.8796, -5.2122) (-68.9359, -5.2586) (-68.9919, -5.3054) (-69.0477, -5.3526) (-69.1034, -5.4003) (-69.1588, -5.4483) (-69.2141, -5.4968) (-69.2692, -5.5457) (-69.324, -5.5951) (-69.3787, -5.6448) (-69.4331, -5.6949) (-69.4874, -5.7454) (-69.5414, -5.7964) (-69.5953, -5.8477) (-69.6489, -5.8994) (-69.7023, -5.9515) (-69.7556, -6.004) (-69.8086, -6.0569) (-69.8614, -6.1101) (-69.914, -6.1637) (-69.9664, -6.2177) (-70.0186, -6.2721) (-70.0706, -6.3268) (-70.1223, -6.3819) (-70.1636, -6.4263) (-70.1944, -6.4597) (-70.215, -6.4821) (-70.2252, -6.4933) knots 0 0 0 0 0 0 0.01428571 0.02857143 0.04285714 0.05714286 0.07142857 0.08571429 0.1 0.11428571 0.12857143 0.14285714 0.15714286 0.17142857 0.18571429 0.2 0.21428571 0.22857143 0.24285714 0.25714286 0.27142857 0.28571429 0.3 0.31428571 0.32857143 0.34285714 0.35714286 0.37142857 0.38571429 0.4 0.41428571 0.42857143 0.44285714 0.45714286 0.47142857 0.48571429 0.5 0.51428571 0.52857143 0.54285714 0.55714286 0.57142857 0.58571429 0.6 0.61428571 0.62857143 0.64285714 0.65714286 0.67142857 0.68571429 0.7 0.71428571 0.72857143 0.74285714 0.75714286 0.77142857 0.78571429 0.8 0.81428571 0.82857143 0.84285714 0.85714286 0.87142857 0.88571429 0.9 0.91428571 0.92857143 0.94285714 0.95714286 0.97142857 0.98571429 1 1 1 1 1 1
  arc A13 (-70.2252, -6.4933) -> (-69.7321, -8.3338) centre (-45.4614, -0.8441) ccw
  spline S7 degree 5 poles (-69.7321, -8.3338) (-69.7176, -8.3383) (-69.6886, -8.3474) (-69.6452, -8.361) (-69.5873, -8.3788) (-69.5149, -8.4006) (-69.4425, -8.422) (-69.3701, -8.443) (-69.2978, -8.4636) (-69.2254, -8.4837) (-69.153, -8.5034) (-69.0807, -8.5227) (-69.0083, -8.5415) (-68.936, -8.5599) (-68.8637, -8.5779) (-68.7914, -8.5954) (-68.7191, -8.6125) (-68.6469, -8.6291) (-68.5747, -8.6453) (-68.5025, -8.6611) (-68.4303, -8.6763) (-68.3582, -8.6912) (-68.2861, -8.7055) (-68.214, -8.7194) (-68.142, -8.7329) (-68.07, -8.7459) (-67.9981, -8.7584) (-67.9262, -8.7704) (-67.8544, -8.782) (-67.7826, -8.793) (-67.7109, -8.8036) (-67.6392, -8.8137) (-67.5676, -8.8233) (-67.496, -8.8324) (-67.4246, -8.8411) (-67.3532, -8.8492) (-67.2818, -8.8568) (-67.2106, -8.8639) (-67.1394, -8.8704) (-67.0683, -8.8765) (-66.9973, -8.882) (-66.9264, -8.887) (-66.8556, -8.8914) (-66.7849, -8.8953) (-66.7143, -8.8986) (-66.6438, -8.9014) (-66.5734, -8.9036) (-66.5031, -8.9052) (-66.4329, -8.9063) (-66.3629, -8.9068) (-66.293, -8.9067) (-66.2232, -8.9059) (-66.1536, -8.9045) (-66.0842, -8.9023) (-66.0149, -8.8995) (-65.9458, -8.8961) (-65.8768, -8.8921) (-65.808, -8.8875) (-65.7394, -8.8823) (-65.6709, -8.8763) (-65.6026, -8.8696) (-65.5347, -8.8618) (-65.467, -8.853) (-65.3997, -8.8431) (-65.3327, -8.8323) (-65.2658, -8.8208) (-65.1992, -8.8087) (-65.1327, -8.7962) (-65.0665, -8.783) (-65.0007, -8.7684) (-64.9356, -8.7517) (-64.8844, -8.736) (-64.8465, -8.7226) (-64.8215, -8.7129) (-64.809, -8.7078) knots -1 -1 -1 -1 -1 -1 -0.98571429 -0.97142857 -0.95714286 -0.94285714 -0.92857143 -0.91428571 -0.9 -0.88571429 -0.87142857 -0.85714286 -0.84285714 -0.82857143 -0.81428571 -0.8 -0.78571429 -0.77142857 -0.75714286 -0.74285714 -0.72857143 -0.71428571 -0.7 -0.68571429 -0.67142857 -0.65714286 -0.64285714 -0.62857143 -0.61428571 -0.6 -0.58571429 -0.57142857 -0.55714286 -0.54285714 -0.52857143 -0.51428571 -0.5 -0.48571429 -0.47142857 -0.45714286 -0.44285714 -0.42857143 -0.41428571 -0.4 -0.38571429 -0.37142857 -0.35714286 -0.34285714 -0.32857143 -0.31428571 -0.3 -0.28571429 -0.27142857 -0.25714286 -0.24285714 -0.22857143 -0.21428571 -0.2 -0.18571429 -0.17142857 -0.15714286 -0.14285714 -0.12857143 -0.11428571 -0.1 -0.08571429 -0.07142857 -0.05714286 -0.04285714 -0.02857143 -0.01428571 0 0 0 0 0 0
  line L9 (-64.809, -8.7078) -> (-63.8852, -8.3329)
  arc A14 (-61.8697, -9.0909) -> (-63.8852, -8.3329) centre (-63.2882, -9.8038) ccw
  arc A15 (-61.8697, -9.0909) -> (-61.5183, -9.7558) centre (-45.4614, -0.8441) ccw
  arc A16 (-62.0273, -11.8481) -> (-61.5183, -9.7558) centre (-62.9064, -10.5262) ccw
  line L10 (-62.0273, -11.8481) -> (-62.8576, -12.4002)
  spline S8 degree 5 poles (-62.8576, -12.4002) (-62.8688, -12.4076) (-62.8909, -12.4228) (-62.9233, -12.4465) (-62.9652, -12.48) (-63.0156, -12.5244) (-63.0647, -12.5705) (-63.1129, -12.6178) (-63.1607, -12.6657) (-63.2082, -12.714) (-63.2554, -12.7627) (-63.3021, -12.812) (-63.3482, -12.8621) (-63.3936, -12.913) (-63.4383, -12.9648) (-63.4823, -13.0173) (-63.5258, -13.0706) (-63.5688, -13.1243) (-63.6114, -13.1786) (-63.6535, -13.2333) (-63.6953, -13.2885) (-63.7366, -13.3442) (-63.7775, -13.4004) (-63.8179, -13.4571) (-63.8578, -13.5143) (-63.8973, -13.5719) (-63.9363, -13.6301) (-63.975, -13.6887) (-64.0132, -13.7477) (-64.051, -13.8071) (-64.0885, -13.8669) (-64.1255, -13.9271) (-64.1621, -13.9877) (-64.1984, -14.0487) (-64.2342, -14.1101) (-64.2696, -14.1719) (-64.3047, -14.234) (-64.3393, -14.2965) (-64.3736, -14.3594) (-64.4075, -14.4226) (-64.441, -14.4862) (-64.4742, -14.5501) (-64.507, -14.6143) (-64.5394, -14.6789) (-64.5714, -14.7438) (-64.603, -14.809) (-64.6343, -14.8746) (-64.6652, -14.9404) (-64.6958, -15.0066) (-64.726, -15.0731) (-64.7558, -15.1399) (-64.7853, -15.207) (-64.8144, -15.2743) (-64.8431, -15.342) (-64.8715, -15.4099) (-64.8995, -15.4782) (-64.9272, -15.5467) (-64.9545, -15.6155) (-64.9815, -15.6845) (-65.0081, -15.7539) (-65.0343, -15.8235) (-65.0602, -15.8933) (-65.0857, -15.9635) (-65.1109, -16.0339) (-65.1357, -16.1045) (-65.1602, -16.1754) (-65.1844, -16.2465) (-65.2081, -16.3179) (-65.2316, -16.3895) (-65.2547, -16.4614) (-65.2774, -16.5335) (-65.2953, -16.5914) (-65.3086, -16.6349) (-65.3174, -16.6639) (-65.3217, -16.6785) knots 0 0 0 0 0 0 0.01428571 0.02857143 0.04285714 0.05714286 0.07142857 0.08571429 0.1 0.11428571 0.12857143 0.14285714 0.15714286 0.17142857 0.18571429 0.2 0.21428571 0.22857143 0.24285714 0.25714286 0.27142857 0.28571429 0.3 0.31428571 0.32857143 0.34285714 0.35714286 0.37142857 0.38571429 0.4 0.41428571 0.42857143 0.44285714 0.45714286 0.47142857 0.48571429 0.5 0.51428571 0.52857143 0.54285714 0.55714286 0.57142857 0.58571429 0.6 0.61428571 0.62857143 0.64285714 0.65714286 0.67142857 0.68571429 0.7 0.71428571 0.72857143 0.74285714 0.75714286 0.77142857 0.78571429 0.8 0.81428571 0.82857143 0.84285714 0.85714286 0.87142857 0.88571429 0.9 0.91428571 0.92857143 0.94285714 0.95714286 0.97142857 0.98571429 1 1 1 1 1 1
  arc A17 (-65.3217, -16.6785) -> (-64.0789, -18.1227) centre (-45.4614, -0.8441) ccw
  spline S9 degree 5 poles (-64.0789, -18.1227) (-64.0638, -18.1205) (-64.0338, -18.1162) (-63.9888, -18.1095) (-63.9289, -18.1005) (-63.8542, -18.0887) (-63.7797, -18.0766) (-63.7054, -18.0641) (-63.6313, -18.0512) (-63.5573, -18.038) (-63.4836, -18.0243) (-63.41, -18.0103) (-63.3367, -17.9959) (-63.2635, -17.9811) (-63.1906, -17.9659) (-63.1179, -17.9503) (-63.0453, -17.9344) (-62.973, -17.918) (-62.9009, -17.9012) (-62.8291, -17.8841) (-62.7574, -17.8666) (-62.686, -17.8486) (-62.6148, -17.8303) (-62.5438, -17.8115) (-62.4731, -17.7924) (-62.4026, -17.7729) (-62.3324, -17.7529) (-62.2624, -17.7326) (-62.1927, -17.7118) (-62.1232, -17.6907) (-62.054, -17.6691) (-61.985, -17.6471) (-61.9163, -17.6247) (-61.8479, -17.6018) (-61.7798, -17.5786) (-61.7119, -17.5549) (-61.6444, -17.5308) (-61.5771, -17.5063) (-61.5101, -17.4813) (-61.4435, -17.4559) (-61.3771, -17.4301) (-61.311, -17.4038) (-61.2453, -17.3771) (-61.1799, -17.3499) (-61.1149, -17.3222) (-61.0502, -17.2941) (-60.9858, -17.2656) (-60.9217, -17.2366) (-60.8581, -17.2071) (-60.7947, -17.1772) (-60.7318, -17.1467) (-60.6693, -17.1158) (-60.6072, -17.0843) (-60.5456, -17.0522) (-60.4844, -17.0197) (-60.4236, -16.9866) (-60.3632, -16.9531) (-60.3032, -16.919) (-60.2436, -16.8845) (-60.1845, -16.8495) (-60.1259, -16.8138) (-60.0681, -16.7773) (-60.011, -16.74) (-59.9546, -16.7019) (-59.8989, -16.663) (-59.8437, -16.6237) (-59.7888, -16.5839) (-59.7344, -16.5438) (-59.6804, -16.5031) (-59.6275, -16.4615) (-59.5761, -16.4182) (-59.5367, -16.3818) (-59.5084, -16.3533) (-59.4901, -16.3337) (-59.4811, -16.3237) knots -1 -1 -1 -1 -1 -1 -0.98571429 -0.97142857 -0.95714286 -0.94285714 -0.92857143 -0.91428571 -0.9 -0.88571429 -0.87142857 -0.85714286 -0.84285714 -0.82857143 -0.81428571 -0.8 -0.78571429 -0.77142857 -0.75714286 -0.74285714 -0.72857143 -0.71428571 -0.7 -0.68571429 -0.67142857 -0.65714286 -0.64285714 -0.62857143 -0.61428571 -0.6 -0.58571429 -0.57142857 -0.55714286 -0.54285714 -0.52857143 -0.51428571 -0.5 -0.48571429 -0.47142857 -0.45714286 -0.44285714 -0.42857143 -0.41428571 -0.4 -0.38571429 -0.37142857 -0.35714286 -0.34285714 -0.32857143 -0.31428571 -0.3 -0.28571429 -0.27142857 -0.25714286 -0.24285714 -0.22857143 -0.21428571 -0.2 -0.18571429 -0.17142857 -0.15714286 -0.14285714 -0.12857143 -0.11428571 -0.1 -0.08571429 -0.07142857 -0.05714286 -0.04285714 -0.02857143 -0.01428571 0 0 0 0 0 0
  line L11 (-59.4811, -16.3237) -> (-58.8114, -15.585)
  arc A18 (-56.6667, -15.3936) -> (-58.8114, -15.585) centre (-57.6353, -16.6513) ccw
  arc A19 (-56.6667, -15.3936) -> (-56.0616, -15.8401) centre (-45.4614, -0.8441) ccw
  arc A20 (-55.6124, -17.946) -> (-56.0616, -15.8401) centre (-56.9779, -17.1365) ccw
  line L12 (-55.6124, -17.946) -> (-56.1208, -18.8037)
  spline S10 degree 5 poles (-56.1208, -18.8037) (-56.1277, -18.8152) (-56.141, -18.8385) (-56.1599, -18.874) (-56.1831, -18.9223) (-56.2093, -18.9842) (-56.2335, -19.047) (-56.2565, -19.1106) (-56.2788, -19.1744) (-56.3006, -19.2386) (-56.322, -19.3029) (-56.3426, -19.3676) (-56.3624, -19.4327) (-56.3813, -19.4983) (-56.3991, -19.5643) (-56.4159, -19.6308) (-56.432, -19.6976) (-56.4474, -19.7647) (-56.4622, -19.8321) (-56.4765, -19.8997) (-56.4902, -19.9675) (-56.5032, -20.0356) (-56.5157, -20.104) (-56.5275, -20.1726) (-56.5386, -20.2414) (-56.5492, -20.3105) (-56.5591, -20.3799) (-56.5685, -20.4494) (-56.5774, -20.5191) (-56.5857, -20.5891) (-56.5935, -20.6592) (-56.6007, -20.7295) (-56.6074, -20.8) (-56.6136, -20.8707) (-56.6192, -20.9416) (-56.6243, -21.0126) (-56.629, -21.0838) (-56.6331, -21.1551) (-56.6367, -21.2267) (-56.6398, -21.2983) (-56.6424, -21.3701) (-56.6446, -21.4421) (-56.6462, -21.5142) (-56.6474, -21.5864) (-56.6481, -21.6588) (-56.6483, -21.7313) (-56.648, -21.804) (-56.6473, -21.8767) (-56.6461, -21.9496) (-56.6445, -22.0226) (-56.6424, -22.0957) (-56.6398, -22.1689) (-56.6368, -22.2422) (-56.6333, -22.3157) (-56.6294, -22.3892) (-56.6251, -22.4628) (-56.6203, -22.5366) (-56.615, -22.6104) (-56.6093, -22.6843) (-56.6032, -22.7583) (-56.5967, -22.8324) (-56.5897, -22.9066) (-56.5823, -22.9809) (-56.5744, -23.0552) (-56.5662, -23.1296) (-56.5575, -23.2041) (-56.5483, -23.2787) (-56.5388, -23.3533) (-56.5288, -23.428) (-56.5184, -23.5028) (-56.5076, -23.5776) (-56.4987, -23.6375) (-56.4918, -23.6825) (-56.4871, -23.7125) (-56.4847, -23.7275) knots 0 0 0 0 0 0 0.01428571 0.02857143 0.04285714 0.05714286 0.07142857 0.08571429 0.1 0.11428571 0.12857143 0.14285714 0.15714286 0.17142857 0.18571429 0.2 0.21428571 0.22857143 0.24285714 0.25714286 0.27142857 0.28571429 0.3 0.31428571 0.32857143 0.34285714 0.35714286 0.37142857 0.38571429 0.4 0.41428571 0.42857143 0.44285714 0.45714286 0.47142857 0.48571429 0.5 0.51428571 0.52857143 0.54285714 0.55714286 0.57142857 0.58571429 0.6 0.61428571 0.62857143 0.64285714 0.65714286 0.67142857 0.68571429 0.7 0.71428571 0.72857143 0.74285714 0.75714286 0.77142857 0.78571429 0.8 0.81428571 0.82857143 0.84285714 0.85714286 0.87142857 0.88571429 0.9 0.91428571 0.92857143 0.94285714 0.95714286 0.97142857 0.98571429 1 1 1 1 1 1
  arc A21 (-56.4847, -23.7275) -> (-54.7383, -24.4894) centre (-45.4614, -0.8441) ccw